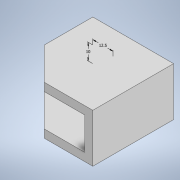
# Autodesk Inventor part: flat_corner
Saved by Autodesk Inventor 2022 (Build 260153000, 153)
## iProperties
Created: 2022-06-12
Part Number: flat_corner
Material: ABS Plastic
Document SubType Name: Modeling
Designer: logic
Density: 1.06 g/cm^3
Appearance: Orange-Red
Author: logic
Autodesk Inventor part; units mm, degrees
ref_plane "YZ Plane" through (0, 0, 0) normal (1, 0, 0) x (0, 1, 0)
ref_plane "XZ Plane" through (0, 0, 0) normal (0, 1, 0) x (-1, 0, 0)
ref_plane "XY Plane" through (0, 0, 0) normal (0, 0, 1) x (1, 0, 0)
sketch "Sketch1" plane through (0, 0, 0) normal (0, 1, 0) x (-1, 0, 0)
  line L0 (-10, 10) -> (10, 10)
  line L1 (10, 10) -> (10, -10)
  line L2 (10, -10) -> (-10, -10)
  line L3 (-10, -10) -> (-10, 10)
  point P0 (0, 0)
  dimension "d0" = 20
  dimension "d1" = 20
  dimension "d2" = 10
  dimension "d3" = 10
  constraints: 8 end point, 2 parallel, 1 horizontal, 1 perpendicular
  measures "d0" distance of L1.end L2.end
  measures "d1" distance of L0.end L1.end
  measures "d2" distance from line of point (0, 0) L3
  measures "d3" distance from line of point (0, 0) L0
extrude "Extrusion1" add sketch "Sketch1" along normal blind 20
sketch "Sketch2" plane through (0, 0, 0) normal (0, -1, 0) x (1, 0, 0)
  line L0 (15, -15) -> (-35, -15)
  line L1 (-35, -15) -> (-35, 15)
  line L2 (-35, 15) -> (-15, 35)
  line L3 (-15, 35) -> (15, 35)
  line L4 (15, 35) -> (15, -15)
  line L5 (10, -10) -> (-10, -10) projected
  line L6 (10, 10) -> (10, -10) projected
  point P0 (0, 0)
  dimension "d6" = 5
  dimension "d7" = 5
  dimension "d8" = 135
  dimension "d9" = 30
  dimension "d10" = 30
  dimension "d11" = 50
  constraints: 10 end point, 1 horizontal, 1 parallel, 1 perpendicular, 1 vertical
  measures "d6" distance between parallel lines of L5 L0
  measures "d7" distance between parallel lines of L6 L4
  measures "d8" angle of L2 L3
  measures "d9" distance of L2.end L3.end
  measures "d10" distance of L0.end L1.end
  measures "d11" distance of L3.end L0.start
extrude "Extrusion2" add sketch "Sketch2" along normal blind 5
sketch "Sketch4" plane through (0, 0, 0) normal (0, 1, 0) x (1, 0, 0)
  point P0 (0, 0)
sketch "Sketch5" plane through (0, 0, 0) normal (0, 1, 0) x (1, 0, 0)
  point P0 (0, 0)
sketch "Sketch6" plane through (0, 0, 0) normal (0, 1, 0) x (1, 0, 0)
  line L0 (10, -30) -> (10, 10)
  line L1 (10, 10) -> (-30, 10)
  line L2 (-30, 10) -> (-30, 15)
  line L3 (-30, 15) -> (15, 15)
  line L4 (15, 15) -> (15, -30)
  line L5 (15, -30) -> (10, -30)
  line L6 (15, -35) -> (-15, -35) projected
  line L7 (-35, -15) -> (-35, 15) projected
  point P0 (0, 0)
  dimension "d18" = 5
  dimension "d21" = 5
  constraints: 12 end point, 5 perpendicular, 2 coincident, 1 vertical
  measures "d18" distance between parallel lines of L5 L6
  measures "d21" distance between parallel lines of L2 L7
extrude "Extrusion4" add sketch "Sketch6" along normal blind 20
sketch "Sketch7" plane through (0, 20, 0) normal (0, 1, 0) x (1, 0, 0)
  line L0 (-10, 10) -> (-30, 10) projected
  line L1 (-30, 10) -> (-30, 15) projected
  line L2 (-35, 15) -> (-30, 15) projected
  line L3 (-35, -15) -> (-35, 15) projected
  line L4 (-15, -35) -> (-35, -15) projected
  line L5 (15, -35) -> (-15, -35) projected
  line L6 (15, -30) -> (15, -35) projected
  line L7 (15, -30) -> (10, -30) projected
  line L8 (10, -30) -> (10, -10) projected
  line L9 (-10, -10) -> (10, -10) projected
  line L10 (-10, 10) -> (-10, -10) projected
  line L11 (-10, 10) -> (-10, -10) projected
  line L12 (-10, -10) -> (10, -10) projected
  line L13 (10, -10) -> (10, -30) projected
  line L14 (10, -30) -> (15, -30) projected
  line L15 (15, -30) -> (15, 15) projected
  line L16 (15, 15) -> (-30, 15) projected
  line L17 (-30, 15) -> (-30, 10) projected
  line L18 (-30, 10) -> (-10, 10) projected
  line L19 (15, -35) -> (-15, -35)
  line L20 (-15, -35) -> (-35, -15)
  line L21 (-35, -15) -> (-35, 15)
  line L22 (-35, 15) -> (15, 15)
  line L23 (15, 15) -> (15, -35)
  point P0 (0, 0)
  constraints: 11 end point, 3 perpendicular, 1 horizontal
extrude "Extrusion5" add sketch "Sketch7" along normal blind 5
sketch "Sketch8" plane through (10, 0, 30) normal (0, 0, 1) x (1, 0, 0)
  line L0 (5, 20) -> (0, 20)
  line L1 (0, 20) -> (0, 0)
  line L2 (0, 0) -> (5, 0)
  line L3 (5, 0) -> (5, 20)
  point P0 (-10, 0)
  constraints: 8 end point, 2 coincident, 2 parallel, 1 horizontal, 1 perpendicular
extrude "Extrusion6" add sketch "Sketch8" along normal blind 5
sketch "Sketch9" plane through (-30, 0, -15) normal (-1, 0, 0) x (0, 0, 1)
  line L0 (5, 20) -> (0, 20)
  line L1 (0, 20) -> (0, 0)
  line L2 (0, 0) -> (5, 0)
  line L3 (5, 0) -> (5, 20)
  point P0 (15, 0)
  constraints: 8 end point, 2 coincident, 2 parallel, 1 horizontal, 1 perpendicular
extrude "Extrusion7" add sketch "Sketch9" along normal blind 5
sketch "Sketch13" plane through (15, -5, -15) normal (0, 0, -1) x (-1, 0, 0)
  line L0 (25, 5) -> (25, 25) projected
  line L1 (50, 25) -> (25, 25) projected
  line L2 (50, 5) -> (50, 25) projected
  line L3 (25, 5) -> (50, 5) projected
  line L4 (37.5, 5) -> (50, 5) construction
  line L5 (50, 5) -> (50, 15) construction
  line L6 (50, 15) -> (37.5, 15) construction
  line L7 (37.5, 15) -> (37.5, 5) construction
  point P0 (15, 5)
  dimension "d32" = 12.5
  dimension "d33" = 10
  constraints: 8 end point, 2 parallel, 1 coincident, 1 horizontal, 1 perpendicular
  measures "d32" distance of L6.end L5.end
  measures "d33" distance of L2.start L5.end
sketch "Sketch14" plane through (15, -5, 35) normal (1, 0, 0) x (0, 0, -1)
  line L0 (25, 5) -> (25, 25) projected
  line L1 (0, 5) -> (25, 5) projected
  line L2 (0, 25) -> (0, 5) projected
  line L3 (25, 25) -> (0, 25) projected
  line L4 (12.5, 15) -> (0, 15) construction
  line L5 (0, 15) -> (0, 25) construction
  line L6 (0, 25) -> (12.5, 25) construction
  line L7 (12.5, 25) -> (12.5, 15) construction
  point P0 (35, 5)
  dimension "d34" = 12.5
  dimension "d35" = 10
  constraints: 8 end point, 2 parallel, 1 coincident, 1 horizontal, 1 perpendicular
  measures "d34" distance of L2.start L6.end
  measures "d35" distance of L2.start L4.end
hole "Hole1" at (15, 10, 22.5) direction (-1, 0, 0) diameter 3.4 end through all counterbore diameter 6.5 counterbore depth 3 clearance for "Socket Head Cap Screw ISO 4762" size "M3" standard "ISO"
hole "Hole2" at (-22.5, 10, -15) direction (0, 0, 1) diameter 3.4 end through all counterbore diameter 6.5 counterbore depth 3 clearance for "Socket Head Cap Screw ISO 4762" size "M3" standard "ISO"
fillet "Fillet1" radius 10 1 edges at (15, 10, -15)
fillet "Fillet2" radius 5 6 edges at (12.0711, -5, -12.0711) (15, -5, 15) (-15, -5, -15) (12.0711, 25, -12.0711) (15, 25, 15) (-15, 25, -15)
fillet "Fillet3" radius 2 12 edges at (-25, 25, 25) (13.5355, 23.5355, 35) (15, 10, 35) (13.5355, -3.5355, 35) (-2.5, -5, 35) (-2.5, 25, 35) (-25, -5, 25) (-35, -3.5355, -13.5355) (-35, 10, -15) (-35, 23.5355, -13.5355) (-35, 25, 2.5) (-35, -5, 2.5)
body "Solid1"
